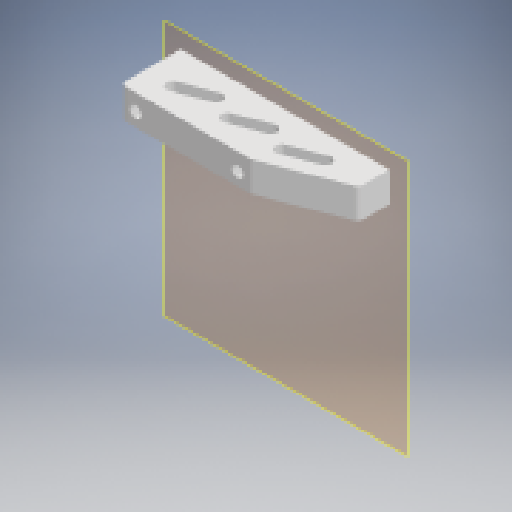
# Autodesk Inventor part: PCB-LNA_Print_CPY
Saved by Autodesk Inventor 2025.2 (Build 292293000, 293)
## iProperties
Created: 2024-12-02
Part Number: PCB-LNA_Print_CPY
Material: Generic
Document SubType Name: Modeling
Designer: Paul Linke
Density: 1 g/cm^3
Appearance: Default
Author: Paul Linke
Autodesk Inventor part; units mm, degrees
ref_plane "YZ Plane" through (0, 0, 0) normal (1, 0, 0) x (0, 1, 0)
ref_plane "XZ Plane" through (0, 0, 0) normal (0, 1, 0) x (-1, 0, 0)
ref_plane "XY Plane" through (0, 0, 0) normal (0, 0, 1) x (1, 0, 0)
ref_plane "Work Plane1" through (0, 0, 0) normal (0, 0, 1) x (1, 0, 0)
sketch "Sketch1" plane through (0, 0, 0) normal (0, 0, 1) x (1, 0, 0)
  circle A0 centre (132.5, -74.5) radius 1.45 projected
  circle A1 centre (177, -74.5) radius 1.45 projected
  line L0 (128.75, -70.75) -> (180.75, -70.75)
  line L1 (180.75, -70.75) -> (180.75, -78.25)
  line L2 (180.75, -78.25) -> (128.75, -78.25)
  line L3 (128.75, -78.25) -> (128.75, -70.75)
  circle A2 centre (132.5, -74.5) radius 1.45
  circle A3 centre (177, -74.5) radius 1.45
  point P0 (0, 0)
  dimension "d0" = 3.75
  dimension "d1" = 3.75
  dimension "d2" = 3.75
  dimension "d3" = 3.75
  constraints: 8 end point, 2 centre point, 2 coincident, 2 concentric, 2 parallel, 1 horizontal, 1 perpendicular
  measures "d0" distance from line of L1 A1.centre
  measures "d1" distance from line of L2 A1.centre
  measures "d2" distance from line of L0 A0.centre
  measures "d3" distance from line of L3 A0.centre
extrude "Extrusion1" add sketch "Sketch1" along normal blind 15
sketch "Sketch2" plane through (0, 0, 15) normal (0, 0, 1) x (1, 0, 0)
  line L0 (128.75, -78.25) -> (180.75, -78.25) projected
  line L1 (180.75, -78.25) -> (180.75, -70.75) projected
  line L2 (180.75, -70.75) -> (128.75, -70.75) projected
  line L3 (128.75, -70.75) -> (128.75, -78.25) projected
  circle A0 centre (177, -74.5) radius 1.45 projected
  circle A1 centre (132.5, -74.5) radius 1.45 projected
  circle A2 centre (177, -74.5) radius 1.45
  circle A3 centre (132.5, -74.5) radius 1.45
  point P0 (0, 0)
  constraints: 2 centre point, 2 coincident, 1 concentric
extrude "Extrusion2" add sketch "Sketch2" against normal blind 8 contours A1
sketch "Sketch4" plane through (0, 0, 15) normal (0, 0, 1) x (1, 0, 0)
  circle A0 centre (177, -74.5) radius 1.45 projected
  circle A1 centre (177, -74.5) radius 1.45
  point P0 (0, 0)
  constraints: 1 centre point, 1 coincident, 1 concentric
extrude "Extrusion3" add sketch "Sketch4" against normal blind 8
sketch "Sketch5" plane through (128.75, -70.75, 0) normal (0, 1, 0) x (1, 0, 0)
  line L0 (52, 0) -> (0, 0) projected
  line L1 (0, 0) -> (0, -15) projected
  line L2 (52, -15) -> (0, -15) projected
  line L3 (52, 0) -> (52, -15) projected
  line L4 (52, -15) -> (0, -15)
  line L5 (0, -15) -> (0, 0)
  line L6 (0, 0) -> (52, 0)
  line L7 (52, 0) -> (52, -15)
  line L8 (52, -15) -> (0, -15) projected
  line L9 (27.805, -15) -> (30.495, -15) projected
  line L10 (30.495, -16) -> (27.805, -16) projected
  line L11 (30.495, -16) -> (30.495, -15)
  line L12 (27.805, -16) -> (27.805, -15)
  line L13 (0, -15) -> (52, -15) projected
  line L14 (32.545, -15) -> (52, -7.5)
  line L15 (52, 0) -> (52, -15) projected
  line L16 (41.9691, -6) -> (34.1871, -9) construction
  line L17 (42.5086, -7.3996) -> (34.7266, -10.3996)
  line L18 (33.6475, -7.6004) -> (41.4295, -4.6004)
  arc A0 (42.5086, -7.3996) -> (41.4295, -4.6004) centre (41.9691, -6) ccw
  arc A1 (33.6475, -7.6004) -> (34.7266, -10.3996) centre (34.1871, -9) ccw
  line L19 (20.0475, -7.6004) -> (27.8295, -4.6004)
  arc A2 (20.0475, -7.6004) -> (21.1266, -10.3996) centre (20.5871, -9) ccw
  line L20 (28.9086, -7.3996) -> (21.1266, -10.3996)
  arc A3 (28.9086, -7.3996) -> (27.8295, -4.6004) centre (28.3691, -6) ccw
  line L21 (-13.6, 0) -> (38.4, 0)
  line L22 (6.4475, -7.6004) -> (14.2295, -4.6004)
  arc A4 (6.4475, -7.6004) -> (7.5266, -10.3996) centre (6.9871, -9) ccw
  line L23 (15.3086, -7.3996) -> (7.5266, -10.3996)
  arc A5 (15.3086, -7.3996) -> (14.2295, -4.6004) centre (14.7691, -6) ccw
  line L24 (-27.2, 0) -> (24.8, 0)
  point P0 (-128.75, 0)
  point P1 (38.0781, -7.5)
  point P2 (52, -7.5)
  point P3 (32.545, -15)
  dimension "d15" = 2.05
  dimension "d21" = 6
  dimension "d22" = 6
  dimension "d23" = 1.5
  dimension "d26" = 13.6
  constraints: 34 end point, 12 point on circle, 6 centre point, 4 parallel, 4 tangent, 2 horizontal, 2 midpoint, 2 vertical, 1 perpendicular, 1 point on line, 26 other
  measures "d15" distance of L9.end L14.start
  measures "d21" distance from line of L0 L16.start
  measures "d22" distance from line of L2 L16.end
  measures "d23" radius of A1
  measures "d26" distance of L18.start L19.start
sketch "Sketch6" plane through (0, 0, 15) normal (0, 0, 1) x (1, 0, 0)
  circle A0 centre (132.5, -74.5) radius 1.45 projected
  line L0 (128.75, -78.25) -> (180.75, -78.25) projected
  line L1 (180.75, -78.25) -> (180.75, -70.75) projected
  line L2 (180.75, -70.75) -> (128.75, -70.75) projected
  line L3 (128.75, -70.75) -> (128.75, -78.25) projected
  circle A1 centre (132.499, -74.9265) radius 1.45
  point P0 (0, 0)
  point P1 (132.5, -74.5)
  dimension "d10" = 2.9
  dimension "d14" = 0.4265
  constraints: 1 centre point
  measures "d10" diameter of A1
  measures "d14" distance of A1.centre A0.centre
extrude "Extrusion4" cut sketch "Sketch6" against normal blind 7 contours A1 A0 | A0 A1 picked at (132.385, -75.1117) picked at (132.6881, -76.0727)
extrude "Extrusion5" cut sketch "Sketch5" against normal blind 8 contours L3 L2 L14 | L17 A1 L18 A0 | L19 A3 L20 A2 | L22 A5 L23 A4
fillet "Fillet1" radius 1.5 3 edges at (180.75, -74.5, 7.5) (161.295, -74.5, 15) (128.75, -74.5, 15)
sketch "Sketch8" plane through (0, 0, 15) normal (0, 0, 1) x (1, 0, 0)
  circle A0 centre (157.9, -75.0575) radius 1.345
  ellipse E0 centre (158.6032, -73.9122) end of major axis (157.4109, -73.2898) minor radius 1.3427 projected
  point P0 (0, 0)
  constraints: 1 centre point, 2 other
extrude "Extrusion7" cut sketch "Sketch8" against normal blind 6.5 contours A0 E0 | A0 E0 picked at (158.3944, -74.3129) picked at (159.1018, -73.1783)
body "Solid1"
